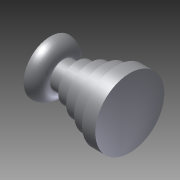
# Autodesk Inventor part: lesson4
Saved by Autodesk Inventor 2011 SP1 (Build 150282100, 282)
## iProperties
Created: 2011-10-08
Part Number: lesson4
Document SubType Name: Modeling
Designer: Kevin
Density: 1 g/cm^3
Author: Kevin
Autodesk Inventor part; units mm, degrees
ref_plane "YZ Plane" through (0, 0, 0) normal (1, 0, 0) x (0, 1, 0)
ref_plane "XZ Plane" through (0, 0, 0) normal (0, 1, 0) x (-1, 0, 0)
ref_plane "XY Plane" through (0, 0, 0) normal (0, 0, 1) x (1, 0, 0)
sketch "Sketch1" plane through (0, 0, 0) normal (0, 0, 1) x (1, 0, 0)
  line L0 (-39.4611, 5.2335) -> (45.3293, 5.2335) construction
  line L1 (28.8024, 5.2335) -> (28.8024, 18.2335)
  line L2 (28.8024, 18.2335) -> (23.8024, 18.2335)
  line L3 (23.8024, 18.2335) -> (23.8024, 16.2335)
  line L4 (23.8024, 16.2335) -> (18.8024, 16.2335)
  line L5 (18.8024, 16.2335) -> (18.8024, 14.2335)
  line L6 (18.8024, 14.2335) -> (13.8024, 14.2335)
  line L7 (13.8024, 14.2335) -> (13.8024, 12.2335)
  line L8 (13.8024, 12.2335) -> (8.8024, 12.2335)
  line L9 (8.8024, 12.2335) -> (8.8024, 10.2335)
  line L10 (8.8024, 10.2335) -> (3.8024, 10.2335)
  arc A0 (3.8024, 10.2335) -> (-1.1976, 15.2335) centre (-1.1976, 10.2335) ccw
  line L11 (-1.1976, 10.2335) -> (-1.1976, 5.2335)
  line L12 (-1.1976, 10.2335) -> (-1.1976, 15.2335)
  line L13 (-1.1976, 5.2335) -> (28.8024, 5.2335)
  point P0 (0, 0)
  dimension "d2" = 5
  dimension "d3" = 5
  dimension "d4" = 5
  dimension "d5" = 5
  dimension "d7" = 5
  dimension "d8" = 2
  dimension "d9" = 2
  dimension "d10" = 2
  dimension "d11" = 2
  dimension "d12" = 10
  constraints: 28 end point, 7 parallel, 4 perpendicular, 2 point on circle, 2 point on line, 1 centre point, 1 collinear, 1 horizontal
  measures "d2" distance of L1.end L2.end
  measures "d3" distance of L3.end L4.end
  measures "d4" distance of L5.end L6.end
  measures "d5" distance of L7.end L8.end
  measures "d7" distance between parallel lines of L0 L10
  measures "d8" distance of L8.end L9.end
  measures "d9" distance of L6.end L7.end
  measures "d10" distance of L4.end L5.end
  measures "d11" distance of L2.end L3.end
  measures "d12" diameter of A0
revolve "Revolution1" add sketch "Sketch1" angle 360 about axis through (-39.4611, 5.2335, 0) along (1, 0, 0)
body "Solid1"
